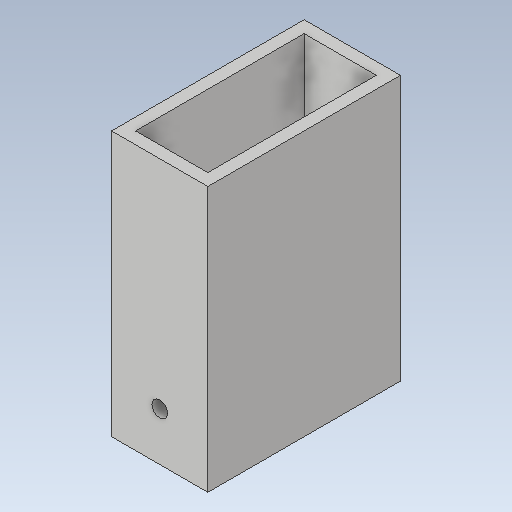
# Autodesk Inventor part: 2x1 2in Alluminum Block.ver1-1111-2019
Saved by Autodesk Inventor 2020 (Build 240168000, 168)
## iProperties
Created: 2019-10-10
Part Number: 2x1 2in Alluminum Block.ver1-1111-2019
Material: Generic
Document SubType Name: Modeling
Designer: JMHal
Density: 1 g/cm^3
Appearance: Default
Author: JMHal
Autodesk Inventor part; units mm, degrees
ref_plane "YZ Plane" through (0, 0, 0) normal (1, 0, 0) x (0, 1, 0)
ref_plane "XZ Plane" through (0, 0, 0) normal (0, 1, 0) x (-1, 0, 0)
ref_plane "XY Plane" through (0, 0, 0) normal (0, 0, 1) x (1, 0, 0)
sketch "Sketch1" plane through (0, 0, 0) normal (0, 1, 0) x (-1, 0, 0)
  line L0 (0, 0) -> (25.4, 0)
  line L1 (25.4, 0) -> (25.4, -50.8)
  line L2 (25.4, -50.8) -> (0, -50.8)
  line L3 (0, -50.8) -> (0, 0)
  line L4 (3.175, -47.625) -> (22.225, -47.625)
  line L5 (22.225, -47.625) -> (22.225, -3.175)
  line L6 (22.225, -3.175) -> (3.175, -3.175)
  line L7 (3.175, -3.175) -> (3.175, -47.625)
  dimension "d0" = 50.8
  dimension "d1" = 25.4
  dimension "d2" = 3.175
  constraints: 16 end point, 4 parallel, 2 perpendicular, 1 horizontal, 3 other
  measures "d0" distance of L0.end L1.end
  measures "d1" distance of L1.end L2.end
  measures "d2" distance between parallel lines of L2 L4
extrude "Extrusion1" add sketch "Sketch1" along normal blind 50.8
sketch "Sketch2" plane through (0, 50.8, 0) normal (0, 1, 0) x (1, 0, 0)
  line L0 (-3.175, 47.625) -> (-3.175, 3.175) projected
  line L1 (-3.175, 3.175) -> (-22.225, 3.175) projected
  line L2 (-22.225, 3.175) -> (-22.225, 47.625) projected
  line L3 (-22.225, 47.625) -> (-3.175, 47.625) projected
  line L4 (-25.4, 0) -> (0, 0) projected
  line L5 (0, 0) -> (0, 50.8) projected
  line L6 (0, 50.8) -> (-25.4, 50.8) projected
  line L7 (-25.4, 50.8) -> (-25.4, 0) projected
extrude "Extrusion2" add sketch "Sketch2" along normal blind 12.7
sketch "Sketch3" plane through (0, 63.5, 0) normal (0, 1, 0) x (1, 0, 0)
  line L0 (-3.175, 3.175) -> (-22.225, 3.175) projected
  line L1 (-22.225, 3.175) -> (-22.225, 47.625) projected
  line L2 (-22.225, 47.625) -> (-3.175, 47.625) projected
  line L3 (-3.175, 47.625) -> (-3.175, 3.175) projected
  line L4 (-25.4, 0) -> (0, 0) projected
  line L5 (0, 0) -> (0, 50.8) projected
  line L6 (0, 50.8) -> (-25.4, 50.8) projected
  line L7 (-25.4, 50.8) -> (-25.4, 0) projected
extrude "Extrusion3" add sketch "Sketch3" along normal blind 6.35
sketch "Sketch4" plane through (-25.4, 0, 0) normal (0, 0, 1) x (1, 0, 0)
  circle A0 centre (12.7, 12.7) radius 2.0701
  line L0 (25.4, 0) -> (0, 0) projected
  line L1 (25.4, 0) -> (25.4, 69.85) projected
  dimension "d9" = 4.1402
  dimension "d10" = 12.7
  dimension "d11" = 12.7
  constraints: 1 centre point
  measures "d9" diameter of A0
  measures "d10" distance from line of A0.centre L0
  measures "d11" distance from line of A0.centre L1
extrude "Extrusion4" cut sketch "Sketch4" against normal blind 25.4
body "Solid1"
